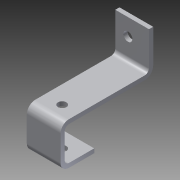
# Autodesk Inventor part: paul mount
Saved by Autodesk Inventor 2013 (Build 170138000, 138)
## iProperties
Created: 2013-02-08
Part Number: paul mount
Material: Aluminum 6061
Document SubType Name: Sheet Metal
Designer: Arpan
Density: 2.71 g/cm^3
Sheet Metal Rule: Default
Mass: 30.4192 g
Surface Area: 83.3473 cm^2
Volume: 11.2248 cm^3
Flat Pattern Width: 2.54 cm
Flat Pattern Length: 14.2195 cm
Flat Pattern Area: 36.1175 cm^2
Sheet Metal Width: 1.000 in
Sheet Metal Length: 5.598 in
Sheet Metal Area: 5.598 in^2
Author: Arpan
Autodesk Inventor part; units mm, degrees
ref_plane "YZ Plane" through (0, 0, 0) normal (1, 0, 0) x (0, 1, 0)
ref_plane "XZ Plane" through (0, 0, 0) normal (0, 1, 0) x (-1, 0, 0)
ref_plane "XY Plane" through (0, 0, 0) normal (0, 0, 1) x (1, 0, 0)
sketch "Sketch1" plane through (0, 0, 0) normal (0, 0, 1) x (1, 0, 0)
  circle A0 centre (9.525, -12.7) radius 3.3782
  line L0 (25.4, 0) -> (0, 0)
  line L1 (0, 0) -> (0, -25.4)
  line L2 (25.4, -25.4) -> (0, -25.4)
  line L3 (25.4, 0) -> (25.4, -25.4)
  dimension "d37" = 25.4
  dimension "d38" = 9.525
extrude "Plate1" add sketch "Sketch1" along normal blind 3.175
sketch "Sketch2" plane through (25.4, -28.575, 6.35) normal (0, -1, 0) x (1, 0, 0)
  line L0 (-25.4, 0) -> (0, 0)
  line L1 (0, 0) -> (0, 57.15)
  line L2 (0, 57.15) -> (-25.4, 57.15)
  line L3 (-25.4, 57.15) -> (-25.4, 0)
  constraints: 6 end point, 1 horizontal, 1 perpendicular, 1 vertical
edge flange "Flange1" height 63.5 angle 90 thickness 3.175 bend radius 3.175 thickness toward (0, -1, 0) relief tear relief width 3.175 relief depth 1.5875 edges at (12.7, -25.4, 3.175) wall of the first edge with corners at (0, -28.575, 6.35) (25.4, -28.575, 6.35) (25.4, -28.575, 63.5) (0, -28.575, 63.5)
bend "Bend1"
corner "Corner1"
sketch "Sketch3" plane through (0, -34.925, 66.675) normal (0, 0, 1) x (1, 0, 0)
  line L0 (25.4, 0) -> (0, 0)
  line L1 (0, 0) -> (0, -19.05)
  line L2 (0, -19.05) -> (25.4, -19.05)
  line L3 (25.4, -19.05) -> (25.4, 0)
  constraints: 6 end point, 1 horizontal, 1 perpendicular, 1 vertical
edge flange "Flange2" height 25.4 angle 90 thickness 3.175 bend radius 3.175 thickness toward (0, 0, 1) relief tear relief width 3.175 relief depth 1.5875 edges at (12.7, -31.75, 63.5) wall of the first edge with corners at (25.4, -34.925, 66.675) (0, -34.925, 66.675) (0, -53.975, 66.675) (25.4, -53.975, 66.675)
bend "Bend2"
corner "Corner2"
sketch "Sketch4" plane through (0, -57.15, 63.5) normal (0, -1, 0) x (1, 0, 0)
  line L0 (25.4, 0) -> (0, 0)
  line L1 (0, 0) -> (0, -19.05)
  line L2 (0, -19.05) -> (25.4, -19.05)
  line L3 (25.4, -19.05) -> (25.4, 0)
  constraints: 6 end point, 1 horizontal, 1 perpendicular, 1 vertical
edge flange "Flange3" height 25.4 angle 90 thickness 3.175 bend radius 3.175 thickness toward (0, -1, 0) relief tear relief width 3.175 relief depth 1.5875 edges at (12.7, -53.975, 66.675) wall of the first edge with corners at (25.4, -57.15, 63.5) (0, -57.15, 63.5) (0, -57.15, 44.45) (25.4, -57.15, 44.45)
bend "Bend3"
corner "Corner3"
sketch "Sketch5" plane through (0, -60.325, 44.45) normal (0, -1, 0) x (1, 0, 0)
  line L0 (-19.05, -30.1625) -> (13.4214, 12.1549)
  line L1 (-19.05, -30.1625) -> (-19.05, 12.1549)
  line L2 (13.4214, 12.1549) -> (-19.05, 12.1549)
  line L3 (-19.05, -30.1625) -> (-8.0357, -30.1625)
  circle A0 centre (13.4214, 12.1549) radius 3.175
  point P0 (0, -44.45)
  dimension "d31" = 53.34
  dimension "d33" = 32.4714
  dimension "d34" = 6.35
  constraints: 8 end point, 1 centre point, 1 coincident, 1 parallel, 1 perpendicular
  measures "d31" distance of L0.start L0.end
  measures "d33" distance of L0.end L1.end
  measures "d34" diameter of A0
extrude "Extrusion1" cut sketch "Sketch5" against normal blind 38.1 contours A0 L2 L0 | L0 L2 A0
equation "\"d1\" = BendReliefWidth"
equation "\"d2\" = BendReliefDepth"
equation "\"d3\" = MinimumRemnant"
equation "\"d4\" = BendRadius"
equation "\"d7\" = BendRadius"
equation "\"d8\" = CornerReliefSize"
equation "\"d9\" = GapSize"
equation "\"d10\" = JacobiRadiusSize"
equation "\"d11\" = BendReliefWidth"
equation "\"d12\" = BendReliefDepth"
equation "\"d13\" = MinimumRemnant"
equation "\"d14\" = BendRadius"
equation "\"d17\" = BendRadius"
equation "\"d18\" = CornerReliefSize"
equation "\"d19\" = GapSize"
equation "\"d20\" = JacobiRadiusSize"
equation "\"d21\" = BendReliefWidth"
equation "\"d22\" = BendReliefDepth"
equation "\"d23\" = MinimumRemnant"
equation "\"d24\" = BendRadius"
equation "\"d27\" = BendRadius"
equation "\"d28\" = CornerReliefSize"
equation "\"d29\" = GapSize"
equation "\"d30\" = JacobiRadiusSize"
equation "\"BendRadius\" = Thickness"
equation "\"BendReliefWidth\" = Thickness"
equation "\"BendReliefDepth\" = 0.5 * Thickness"
equation "\"CornerReliefSize\" = 4 * Thickness"
equation "\"MinimumRemnant\" = 2 * Thickness"
equation "\"TransitionRadius\" = BendRadius"
equation "\"JacobiRadiusSize\" = Thickness"
equation "\"GapSize\" = Thickness"
equation "\"d0\" = BendRadius"
equation "\"Thickness\" = 3.175"
body "Solid1"
